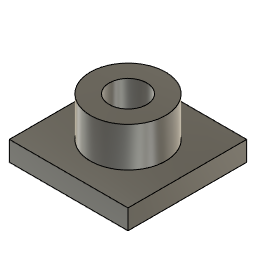
Test v3 (Autodesk Fusion 360 design; units mm, degrees)
Autodesk Fusion 360 part; units mm, degrees
sketch "Sketch2" plane through (0, 0, 0) normal (0, 0, 1) x (1, 0, 0)
  line L0 (0, 0) -> (6, 0)
  line L1 (0, 0) -> (0, 6)
  line L2 (0, 6) -> (6, 6)
  line L3 (6, 6) -> (6, 0)
  circle A0 centre (3, 3) radius 1.9
  circle A1 centre (3, 3) radius 0.95
  dimension "d11" = 6
  dimension "d12" = 6
  dimension "d13" = 6
  dimension "d15" = 3.8
  dimension "d16" = 1.9
  constraint coincident L0.start L1.start
  constraint horizontal L0
  constraint perpendicular L0 L1
  constraint perpendicular L1 L2
  constraint concentric A0 A1
  measures "d11" distance of L0.start L0.end
  measures "d12" distance of L0.start L1.end
  measures "d13" distance of L1.end L2.end
  measures "d15" diameter of A0
  measures "d16" diameter of A1
extrude "Extrude4" add sketch "Sketch2" along normal blind 3 contours A0
extrude "Extrude5" add sketch "Sketch2" along normal blind 1 contours L0 L1 L2 L3
extrude "Extrude6" add sketch "Sketch2" along normal blind 1 contours A1
